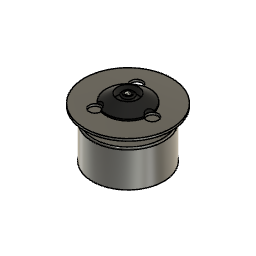
motor3 (Autodesk Fusion 360 design; units mm, degrees)
Autodesk Fusion 360 part; units mm, degrees
sketch "Sketch1" plane through (0, 0, 0) normal (0, 0, 1) x (1, 0, 0)
  circle A0 centre (0, 0) radius 12.2
  dimension "d1" = 24.4
  constraint coincident A0.centre origin
  measures "d1" diameter of A0
extrude "Extrude1" add sketch "Sketch1" along normal blind 12.4 makes body 1
sketch "Sketch2" plane through (0, 0, 0) normal (0, 0, -1) x (1, 0, 0)
  circle A0 centre (0, 0) radius 12.2
  circle A1 centre (0, 0) radius 3
  dimension "d4" = 6
  constraint concentric A0 A1
  measures "d4" diameter of A1
extrude "Extrude2" add sketch "Sketch2" along normal blind 0.6 contours A1 bodies 1
fillet "Fillet1" radius 0.2 1 edges at (-2.797, 1.0848, -0.6) on bodies 1
sketch "Sketch3" plane through (0, 0, 12.4) normal (0, 0, 1) x (-1, 0, 0)
  circle A0 centre (0, 0) radius 12.2
  circle A1 centre (0, 0) radius 1.25
  dimension "d9" = 2.5
  constraint coincident A0.centre A1.centre
  measures "d9" diameter of A1
extrude "Extrude3" cut sketch "Sketch3" against normal blind 12.4 contours A1 bodies 1
copy_body "Body->Comp1" bodies 1 removing the originals makes body 2 in component "motor_body"
sketch "Sketch1 (2)" plane through (0, 0, 0) normal (0, 0, 1) x (1, 0, 0) in component "rotor"
  circle A0 centre (0, 0) radius 1
  dimension "d12" = 2
  constraint coincident A0.centre origin
  measures "d12" diameter of A0
extrude "Extrude1'" add sketch "Sketch1 (2)" along normal blind 22.9 separate body makes body 3 in component "rotor"
fillet "Fillet1'" radius 0.5 1 edges at (-11.3744, -4.4117, 12.4) on bodies 2 in component "motor_body"
ref_plane "WorkPlane1" through (0, 0, 16.4) normal (0, 0, 1) x (1, 0, 0) in component "motor_cap"
sketch "Sketch1 (3)" plane through (0, 0, 16.4) normal (0, 0, 1) x (1, 0, 0) in component "motor_cap"
  circle A0 centre (0, 0) radius 14.9
  circle A1 centre (0, 0) radius 1
  dimension "d22" = 29.8
  dimension "d23" = 2
  constraint coincident A0.centre A1.centre
  constraint concentric A0 A1
  measures "d22" diameter of A0
  measures "d23" diameter of A1
extrude "Extrude1''" add sketch "Sketch1 (3)" along normal blind 0.77 separate body makes body 4 in component "motor_cap"
sketch "Sketch1 (4)" plane through (0, 0, 12.4) normal (0, 0, 1) x (-1, 0, 0) in component "motor_body"
  circle A0 centre (0, 0) radius 1.25
  circle A1 centre (0, 0) radius 11.7
  circle A2 centre (0, 0) radius 3.2
  dimension "d26" = 6.4
  constraint concentric A0 A2
  measures "d26" diameter of A2
extrude "Extrude1'''" add sketch "Sketch1 (4)" along normal blind 1 contours A2 bodies 2 in component "motor_body"
sketch "Sketch1 (5)" plane through (0, 0, 17.17) normal (0, 0, 1) x (-1, 0, 0) in component "motor_plastic_cap"
  circle A0 centre (0, 0) radius 1
  circle A1 centre (0, 0) radius 14.9
  circle A2 centre (0, 0) radius 7.475
  dimension "d29" = 14.95
  constraint concentric A0 A2
  measures "d29" diameter of A2
extrude "Extrude1''''" add sketch "Sketch1 (5)" along normal blind 0.5 separate body contours A0 | A2 makes body 5 in component "motor_plastic_cap"
ref_plane "WorkPlane1" through (0, 0, 20.17) normal (0, 0, 1) x (-1, 0, 0) in component "motor_plastic_cap"
sketch "Sketch2 (2)" plane through (0, 0, 20.17) normal (0, 0, 1) x (1, 0, 0) in component "motor_plastic_cap"
  circle A0 centre (0, 0) radius 3.625
  dimension "d33" = 7.25
  constraint coincident A0.centre origin
  measures "d33" diameter of A0
loft "Loft1" add profiles "Sketch2 (2)" section 1 face at (2.1089, -0.7344, 17.67) section 2 on bodies 5 bodies 5 in component "motor_plastic_cap"
sketch "Sketch3 (2)" plane through (0, 0, 20.17) normal (0, 0, 1) x (-1, 0, 0) in component "motor_plastic_cap"
  circle A0 centre (0, 0) radius 3.625
  circle A1 centre (0, 0) radius 2
  dimension "d34" = 4
  constraint concentric A0 A1
  measures "d34" diameter of A1
extrude "Extrude2'" cut sketch "Sketch3 (2)" against normal blind 2.5 bodies 5 in component "motor_plastic_cap"
chamfer "Chamfer1" distance 0.5 angle 45 1 edges at (1.8647, 0.7232, 20.17) on bodies 5 in component "motor_plastic_cap"
extrude "Extrude2''" cut 1 faces at (-0.3296, 0.5031, 22.9) along direction (0, 0, -1) blind 3.68 on bodies 3 bodies 3 in component "rotor"
sketch "Sketch2 (3)" plane through (0, 0, 17.17) normal (0, 0, 1) x (-1, 0, 0) in component "motor_cap"
  circle A0 centre (0, 0) radius 1
  circle A1 centre (0, 0) radius 14.9 construction
  circle A2 centre (0, -8.3) radius 2
  line L0 (0, 0) -> (0, -14.9) construction
  dimension "d40" = 4
  dimension "d41" = 6.6
  constraint coincident A0.centre A1.centre
  constraint coincident A1 L0.end
  constraint vertical L0
  measures "d40" diameter of A2
  measures "d41" distance of A2.centre L0.end
extrude "Extrude2'''" cut sketch "Sketch2 (3)" along normal blind 3 and the other way blind 2 contours A2 bodies 4 in component "motor_cap"
extrude "Extrude3'" cut sketch "Sketch2 (3)" along normal blind 3 and the other way blind 2 contours A2 bodies 5 in component "motor_plastic_cap"
pattern_circular "C-Pattern1" count 3 over 360 about axis through (0, 0, 19.22) along (0, 0, -1) of "Extrude2'''" in component "motor_cap"
pattern_circular "C-Pattern1'" count 3 over 360 about axis through (0, 0, 19.22) along (0, 0, -1) of "Extrude3'" in component "motor_plastic_cap"
component "motor_body" placed x (1, 0, 0) y (0, 1, 0) z (0, 0, 1) at (0, 0, 0)
component "rotor" placed x (1, 0, 0) y (0, 1, 0) z (0, 0, 1) at (0, 0, 0.95)
component "motor_cap" placed x (1, 0, 0) y (0, 1, 0) z (0, 0, 1) at (0, 0, 0)
component "motor_plastic_cap" placed x (1, 0, 0) y (0, 1, 0) z (0, 0, 1) at (0, 0, 0)
equation "d41 = 4.6 mm + 2 mm"
